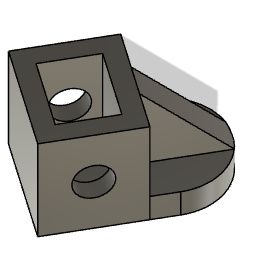
design2 (Autodesk Fusion 360 design; units mm, degrees)
Autodesk Fusion 360 part; units mm, degrees
sketch "Sketch1" plane through (0, 0, 0) normal (1, 0, 0) x (0, 1, 0)
sketch "Sketch1 (2)" plane through (0, 0, 0) normal (0, 0, 1) x (1, 0, 0) in component "Box"
  line L0 (32.0127, 76.0015) -> (-31.9873, 76.0015)
  line L1 (-31.9873, 76.0015) -> (-31.9873, 0.0015)
  line L2 (-31.9873, 0.0015) -> (32.0127, 0.0015)
  line L3 (32.0127, 0.0015) -> (32.0127, 76.0015)
  dimension "d3" = 64
  dimension "d4" = 76
  constraint horizontal L0
  constraint vertical L1
  constraint horizontal L2
  constraint vertical L3
  measures "d3" distance of L0.start L0.end
  measures "d4" distance of L0.start L2.end
extrude "Extrude1" add sketch "Sketch1 (2)" along normal blind 72 makes body 1 in component "Box"
sketch "Sketch2" plane through (0, 0, 72) normal (0, 0, 1) x (-1, 0, 0) in component "Box"
  line L0 (-32.0127, -0.0015) -> (-32.0127, -76.0015)
  line L1 (-32.0127, -76.0015) -> (31.9873, -76.0015)
  line L2 (31.9873, -76.0015) -> (31.9873, -0.0015)
  line L3 (31.9873, -0.0015) -> (-32.0127, -0.0015)
  line L4 (18.8215, -63.0015) -> (-19.1785, -63.0015)
  line L5 (-19.1785, -63.0015) -> (-19.1785, -13.0015)
  line L6 (-19.1785, -13.0015) -> (18.8215, -13.0015)
  line L7 (18.8215, -13.0015) -> (18.8215, -63.0015)
  dimension "d7" = 38
  dimension "d8" = 50
  constraint horizontal L4
  constraint vertical L5
  constraint horizontal L6
  constraint vertical L7
  measures "d7" distance of L4.start L4.end
  measures "d8" distance of L4.start L6.end
extrude "Extrude2" cut sketch "Sketch2" against normal blind 54 contours L4 L5 L6 L7 bodies 1 in component "Box"
sketch "Sketch3" plane through (0, 0.0015, 0) normal (0, -1, 0) x (1, 0, 0) in component "Box"
  line L0 (-31.9873, 0) -> (32.0127, 0)
  line L1 (32.0127, 0) -> (32.0127, 72)
  line L2 (32.0127, 72) -> (-31.9873, 72)
  line L3 (-31.9873, 72) -> (-31.9873, 0)
  circle A0 centre (0.0127, 36) radius 12.5
  line L4 (19.1785, 72) -> (-18.8215, 72)
  dimension "d13" = 25
  dimension "d14" = 32
  measures "d13" diameter of A0
  measures "d14" distance of L3 A0.centre
extrude "Extrude3" cut sketch "Sketch3" against normal blind 75 contours A0 bodies 1 in component "Box"
extrude "Extrude4" cut sketch "Sketch3" against normal blind 140 contours A0 bodies 1 in component "Box"
sketch "Sketch4" plane through (0, 0, 0) normal (0, 0, 1) x (1, 0, 0) in component "Box"
sketch "Sketch1 (3)" plane through (0, 0, 0) normal (0, 0, -1) x (1, 0, 0) in component "Head"
  line L0 (32.0127, -76.0015) -> (32.0127, -0.0015)
  line L1 (32.0127, -0.0015) -> (-31.9873, -0.0015)
  line L2 (-31.9873, -0.0015) -> (-31.9873, -76.0015)
  line L3 (-31.9873, -76.0015) -> (32.0127, -76.0015)
  line L4 (-31.9873, -86.6837) -> (-31.9873, -0.0015) construction
  line L5 (-31.9873, -76.0015) -> (-87.9873, -76.0015)
  line L6 (-87.9873, -76.0015) -> (-87.9873, -0.0015)
  line L7 (-87.9873, -0.0015) -> (-31.9873, -0.0015)
  line L8 (-31.9873, -0.0015) -> (-31.9873, -76.0015)
  line L9 (-31.9873, -49.0015) -> (-87.9873, -49.0015)
  line L10 (-87.9873, -49.0015) -> (-87.9873, -27.0015)
  line L11 (-87.9873, -27.0015) -> (-31.9873, -27.0015)
  line L12 (-31.9873, -27.0015) -> (-31.9873, -49.0015)
  line L13 (-31.9873, -38.0015) -> (-87.9873, -38.0015)
  circle A0 centre (-49.6011, -38.0015) radius 38
  line L14 (-87.9873, -76.0015) -> (-87.9873, -0.0015)
  line L15 (-87.9873, -0.0015) -> (-87.9873, 15) construction
  line L16 (-49.6011, -38.0015) -> (-49.6011, -27.0015) construction
  line L17 (-49.6011, -38.0015) -> (-49.6011, -49.0015) construction
  dimension "d22" = 56
  dimension "d23" = 76
  dimension "d24" = 56
  dimension "d25" = 22
  dimension "d26" = 27
  dimension "d27" = 11
  dimension "d28" = 76
  constraint coincident L2 L4.start
  constraint perpendicular L1 L4
  constraint horizontal L5
  constraint vertical L6
  constraint horizontal L7
  constraint vertical L8
  constraint coincident L2.end L3.start
  constraint horizontal L9
  constraint vertical L10
  constraint horizontal L11
  constraint vertical L12
  constraint coincident L8 L9.start
  constraint midpoint L8 L13.start
  constraint midpoint L10 L13.end
  constraint coincident L1.end L2.start
  constraint coincident L13 A0.centre
  constraint perpendicular L7 L15
  constraint coincident A0.centre L16.start
  constraint coincident L11 L16.end
  constraint perpendicular L11 L16
  constraint coincident L9 L17.end
  constraint perpendicular L13 L17
  measures "d22" distance of L2.end L5.end
  measures "d23" distance of L2.end L1.end
  measures "d24" distance of L9.start L9.end
  measures "d25" distance of L9.start L11.end
  measures "d26" distance of L5 L9
  measures "d27" distance of L9 L13
  measures "d28" diameter of A0
extrude "Extrude1'" add sketch "Sketch1 (3)" against normal blind 18 separate body contours L2 L5 L8 A0 | L2 L7 L8 A0 | L2 L8 L9 A0 | L2 L8 L11 A0 | L2 L8 L9 L12 L13 A0 | L2 L8 L11 L12 L13 A0 makes body 2 in component "Head"
extrude "Extrude2'" add sketch "Sketch1 (3)" against normal blind 72 contours L2 L8 L9 L12 L13 A0 | L2 L8 L11 L12 L13 A0 bodies 2 in component "Head"
sketch "Sketch3 (2)" plane through (0, 49.0015, 0) normal (0, 1, 0) x (-1, 0, 0) in component "Head"
  line L0 (31.9873, 18) -> (85.9742, 18)
  line L1 (85.9742, 18) -> (85.9742, 72)
  line L2 (85.9742, 72) -> (31.9873, 72)
  line L3 (31.9873, 72) -> (31.9873, 18)
  dimension "d34" = 54
  measures "d34" distance of L0 L2
sketch "Sketch4 (2)" plane through (0, 0, 0) normal (0, 0, -1) x (1, 0, 0) in component "Head"
sketch "Sketch10" plane through (0, 0, 72) normal (0, 0, 1) x (-1, 0, 0) in component "Head"
  arc A0 (85.9742, -49.0015) -> (85.9742, -27.0015) centre (49.6011, -38.0015) ccw
  line L0 (85.9742, -27.0015) -> (31.9873, -27.0015)
  line L1 (31.9873, -27.0015) -> (31.9873, -49.0015)
  line L2 (31.9873, -49.0015) -> (85.9742, -49.0015)
sketch "Sketch11" plane through (0, 0, 0) normal (0, 1, 0) x (1, 0, 0) in component "Head"
sketch "Sketch12" plane through (0, 0, 0) normal (0, 1, 0) x (1, 0, 0) in component "Head"
sketch "Sketch13" plane through (0, 0, 18) normal (0, 0, 1) x (-1, 0, 0) in component "Head"
  line L0 (31.9873, -27.0015) -> (85.9742, -27.0015)
  arc A0 (85.9742, -27.0015) -> (49.6011, -0.0015) centre (49.6011, -38.0015) ccw
  line L1 (49.6011, -0.0015) -> (31.9873, -0.0015)
  line L2 (31.9873, -0.0015) -> (31.9873, -27.0015)
sketch "Sketch14" plane through (0, 0, 0) normal (0, 1, 0) x (1, 0, 0) in component "Head"
sketch "Sketch15" plane through (-58.9807, 49.0015, 45) normal (0, 1, 0) x (-1, 0, 0) in component "Head"
sketch "Sketch16" plane through (-58.9807, 49.0015, 45) normal (0, 1, 0) x (-1, 0, 0) in component "Head"
  line L0 (-36.2278, 26.9005) -> (35, 26.9005) construction
  line L1 (-27.3061, -27.1709) -> (62.9932, -27.1709) construction
  constraint horizontal L0
  constraint horizontal L1
sketch "Sketch17" plane through (-58.9807, 49.0015, 45) normal (0, 1, 0) x (-1, 0, 0) in component "Head"
sketch "Sketch18" plane through (-58.9807, 49.0015, 45) normal (0, 1, 0) x (-1, 0, 0) in component "Head"
  line L0 (-31, 31) -> (34.1103, -33.8893)
  line L1 (34.1103, -33.8893) -> (65.2556, -2.638)
  line L2 (65.2556, -2.638) -> (0.1453, 62.2514)
  line L3 (0.1453, 62.2514) -> (-31, 31)
  constraint perpendicular L0 L1
  constraint parallel L0 L2
  constraint parallel L1 L3
extrude "Extrude6" cut sketch "Sketch18" against normal blind 50 bodies 2 in component "Head"
extrude "Extrude3'" [suppressed] in component "Head"
sketch "Sketch6" plane through (0, 0, 0) normal (0, 0, -1) x (1, 0, 0) in component "Head"
  line L0 (-85.9742, -49.0015) -> (-85.9742, -27.0015)
  dimension "d40" = 22
  measures "d40" distance of L0.start L0.end
other "SplitFace1" in component "Head"
other "SplitFace2" in component "Head"
sketch "Sketch7" plane through (-58.9807, 49.0015, 45) normal (0, 1, 0) x (-1, 0, 0) in component "Head"
  line L0 (15, 30) -> (48.8981, 30)
  line L1 (48.8981, 30) -> (48.8981, -9.2148)
  line L2 (48.8981, -9.2148) -> (15, -9.2148)
  line L3 (15, -9.2148) -> (15, 30)
  constraint horizontal L0
  constraint vertical L1
  constraint horizontal L2
  constraint vertical L3
extrude "Extrude4'" [suppressed] in component "Head"
sketch "Sketch8" plane through (-58.9807, 49.0015, 45) normal (0, 1, 0) x (-1, 0, 0) in component "Head"
  circle A0 centre (35, -15) radius 12.6394
extrude "Extrude5" [suppressed] in component "Head"
sketch "Sketch9" plane through (-58.9807, 49.0015, 45) normal (0, 1, 0) x (-1, 0, 0) in component "Head"
  line L0 (-27, 27) -> (27, -27)
  line L1 (27, -27) -> (34, -34) construction
  line L2 (34, -34) -> (44, -44) construction
  constraint parallel L0 L1
  constraint parallel L1 L2
sketch "Sketch2 (2)" plane through (0, 49.0015, 0) normal (0, 1, 0) x (-1, 0, 0) in component "Head"
  line L0 (31.9873, 0) -> (85.9742, 0)
  line L1 (85.9742, 0) -> (85.9742, 54)
  line L2 (85.9742, 54) -> (31.9873, 54)
  line L3 (31.9873, 54) -> (31.9873, 0)
  line L4 (31.9873, 0) -> (87.9873, 0)
  dimension "d33" = 54
  measures "d33" distance of L2 L4
component "Box" placed x (1, 0, 0) y (0, 1, 0) z (0, 0, 1) at (0, 0, 0)
component "Head" placed x (1, 0, 0) y (0, 1, 0) z (0, 0, 1) at (0, 0, 0)
